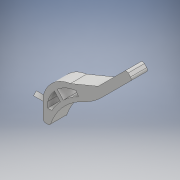
# Autodesk Inventor part: Positioner_Adapter_Der
Saved by Autodesk Inventor 2018 (Build 220112000, 112)
## iProperties
Created: 2017-10-10
Part Number: Positioner_Adapter_Der
Material: Genérico
Document SubType Name: Modeling
Designer: se_ma
Density: 1 g/cm^3
Appearance: Valor por defecto
Author: se_ma
Autodesk Inventor part; units mm, degrees
ref_plane "YZ Plane" through (0, 0, 0) normal (1, 0, 0) x (0, 1, 0)
ref_plane "XZ Plane" through (0, 0, 0) normal (0, 1, 0) x (-1, 0, 0)
ref_plane "XY Plane" through (0, 0, 0) normal (0, 0, 1) x (1, 0, 0)
sketch "Boceto1" plane through (0, 0, 0) normal (0, 1, 0) x (-1, 0, 0)
  line L0 (80, 47.68) -> (80, 52.68)
  line L1 (80, 47.68) -> (80, 22.68)
  line L2 (80, 22.68) -> (75, 22.68)
  line L3 (75, 22.68) -> (71.4886, 22.68)
  line L4 (80, 80) -> (80, 52.68)
  line L5 (20, 72.2842) -> (-29.4975, 121.7816)
  line L6 (20, 72.2842) -> (90, 72.2842) construction
  line L7 (-29.4975, 121.7816) -> (-22.4264, 128.8527)
  line L8 (29.9618, 80) -> (80, 80)
  arc A0 (71.4886, 22.68) -> (20, 72.2842) centre (0, 0) ccw
  line L9 (-22.4264, 128.8527) -> (26.4263, 80)
  line L10 (26.4263, 80) -> (29.9618, 80)
  dimension "d4" = 5
  dimension "d5" = 25
  dimension "d21" = 70
  dimension "d22" = 135
  dimension "d23" = 10
  constraints: 22 end point, 3 horizontal, 2 point on circle, 1 centre point, 1 equal length, 1 parallel, 1 vertical
  measures "d4" distance of L0.start L0.end
  measures "d5" distance of L0.start L1.end
  measures "d21" distance of L5.start L5.end
  measures "d22" angle of L6 L5
  measures "d23" distance of L5.end L7.end
extrude "Extrusión5" add sketch "Boceto1" along normal blind 20
fillet "Empalme3" radius 80 1 edges at (-20, 10, 72.2842)
fillet "Empalme4" radius 3 4 edges at (29.4975, 10, 121.7816) (22.4264, 10, 128.8527) (-71.4886, 10, 22.68) (-80, 10, 22.68)
fillet "Empalme5" radius 30 1 edges at (-80, 10, 80)
chamfer "Chaflán1" distance 20 angle 45 1 edges at (-26.4263, 10, 80)
sketch "Boceto4" plane through (0, 20, 0) normal (0, 1, 0) x (1, 0, 0)
  arc A0 (-69.282, -40) -> (-27.3616, -75.1754) centre (0, 0) ccw
  line L0 (0, 0) -> (-69.282, -40) construction
  line L1 (0, 0) -> (80, 0) construction
  line L2 (0, 0) -> (-27.3616, -75.1754) construction
  line L3 (-69.282, -40) -> (-74.282, -40)
  line L4 (-74.282, -40) -> (-74.282, -47)
  arc A1 (-74.282, -47) -> (-27.3616, -75.1754) centre (-35.8026, -36.0762) ccw
  dimension "d35" = 80
  dimension "d36" = 150
  dimension "d37" = 40
  dimension "d38" = 5
  dimension "d39" = 7
  dimension "d40" = 40
  constraints: 10 end point, 4 point on circle, 2 centre point, 2 horizontal, 1 coincident, 1 equal length, 1 perpendicular
  measures "d35" radius of A0
  measures "d36" angle of L0 L1
  measures "d37" angle of L0 L2
  measures "d38" distance of L0.end L3.end
  measures "d39" distance of L3.end L4.end
  measures "d40" radius of A1
extrude "Extrusión6" cut sketch "Boceto4" against normal blind 20
sketch "Boceto5" plane through (0, 20, 0) normal (0, 1, 0) x (1, 0, 0)
  line L0 (-80, -50) -> (-80, -25.68) projected
  line L1 (-46.4263, -80) -> (-50, -80) projected
  arc A0 (-80, -50) -> (-46.4263, -80) centre (-41.1827, -40.3452) ccw
  arc A1 (-80, -50) -> (-46.4263, -80) centre (-50.0008, -50.2137) ccw
  line L2 (-27.3616, -75.1754) -> (-17.3616, -75.1754) construction
  point P0 (0, 0)
  dimension "d43" = 40
  dimension "d44" = 30
  constraints: 4 point on circle, 2 centre point, 2 end point, 1 horizontal
  measures "d43" radius of A0
  measures "d44" radius of A1
extrude "Extrusión7" cut sketch "Boceto5" against normal blind 20
sketch "Boceto6" plane through (0, 20, 0) normal (0, 1, 0) x (1, 0, 0)
  line L0 (-36.5264, -71.1746) -> (-40.1604, -76.8501)
  line L1 (-40.1604, -76.8501) -> (-29.2954, -83.1239)
  line L2 (-29.2954, -83.1239) -> (-25.1938, -76.0206)
  line L3 (-25.1938, -76.0206) -> (-24.7057, -75.1754)
  line L4 (-24.7057, -75.1754) -> (-35.8148, -69.3243)
  line L5 (-35.8148, -69.3243) -> (-36.5264, -71.1746)
  point P0 (0, 0)
  point P1 (-74.282, -47)
  dimension "d50" = 44.8319
  constraints: 12 end point, 1 perpendicular
  measures "d50" distance of point (-74.282, -47) L0.start
extrude "Extrusión8" add sketch "Boceto6" against normal blind 20
sketch "Boceto7" plane through (0, 20, 0) normal (0, 1, 0) x (1, 0, 0)
  arc A0 (-69.282, -40) -> (-36.5264, -71.1746) centre (0, 0) ccw projected
  line L0 (-69.282, -40) -> (-74.282, -40) projected
  line L1 (-69.282, -40) -> (-69.282, -40)
  arc A1 (-74.282, -47) -> (-39.5521, -75.9) centre (-35.8026, -36.0762) ccw projected
  line L2 (-55.1527, -57.9498) -> (-58.6667, -54.3895)
  line L3 (-66.0968, -62.1963) -> (-58.6667, -54.3895)
  line L4 (-62.599, -65.7738) -> (-55.1527, -57.9498)
  line L5 (-66.0968, -62.1963) -> (-67.4453, -63.6132)
  line L6 (-67.4453, -63.6132) -> (-64.0789, -67.3287)
  line L7 (-64.0789, -67.3287) -> (-62.599, -65.7738)
  constraints: 14 end point, 4 point on circle, 1 collinear, 1 point on line
extrude "Extrusión9" add sketch "Boceto7" against normal blind 20 contours A0 L4 A1 L3 | A1 L7 L6 L5
sketch "Boceto8" plane through (-80, 0, 25.68) normal (-1, 0, 0) x (0, 0, 1)
  line L0 (24.32, 20) -> (24.32, 0) projected
  line L1 (24.32, 20) -> (24.32, 0)
  line L2 (24.32, 0) -> (0, 0) projected
  line L3 (0, 0) -> (0, 20) projected
  line L4 (12.16, 10) -> (22.16, 10) construction
  line L5 (5.0889, 17.0711) -> (6.8567, 18.8388)
  line L6 (19.2311, 2.9289) -> (20.9988, 4.6967)
  line L7 (20.9988, 4.6967) -> (6.8567, 18.8388)
  line L8 (5.0889, 17.0711) -> (3.3212, 15.3033)
  line L9 (3.3212, 15.3033) -> (17.4633, 1.1612)
  line L10 (17.4633, 1.1612) -> (19.2311, 2.9289)
  point P0 (-25.68, 0)
  dimension "d59" = 10
  dimension "d61" = 10
  dimension "d62" = 2.5
  dimension "d63" = 2.5
  constraints: 16 end point, 3 perpendicular, 1 collinear, 1 horizontal
  measures "d59" distance of L4.start L6.start
  measures "d61" distance of L4.start L5.start
  measures "d62" distance of L5.start L5.end
  measures "d63" distance of L5.start L8.end
extrude "Extrusión10" add sketch "Boceto8" along normal blind 13
sketch "Boceto9" plane through (-93, 18.8388, 32.5367) normal (0, 0.7071, 0.7071) x (1, 0, 0)
  line L0 (13, -20) -> (0, -20) projected
  line L1 (0, -20) -> (0, 0) projected
  line L2 (0, -20) -> (0, 0)
  line L3 (3, -10) -> (3, -15)
  line L4 (3, -15) -> (10, -15)
  line L5 (10, -15) -> (10, -5)
  line L6 (10, -5) -> (3, -5)
  line L7 (3, -5) -> (3, -10)
  point P0 (93, 9.6859)
  dimension "d67" = 5
  dimension "d68" = 7
  dimension "d69" = 10
  constraints: 12 end point, 4 perpendicular, 1 point on line, 1 vertical
  measures "d67" distance of L3.start L3.end
  measures "d68" distance of L3.end L4.end
  measures "d69" distance of L4.end L5.end
extrude "Extrusión11" cut sketch "Boceto9" against normal blind 5
